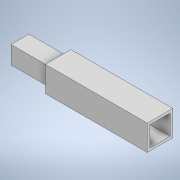
# Autodesk Inventor part: Right Side Piece
Saved by Autodesk Inventor 2022 (Build 260153000, 153)
## iProperties
Created: 2022-01-02
Part Number: Right Side Piece
Material: Generic
Document SubType Name: Modeling
Designer: josephinew
Density: 1 g/cm^3
Appearance: Default
Author: josephinew
Autodesk Inventor part; units mm, degrees
ref_plane "YZ Plane" through (0, 0, 0) normal (1, 0, 0) x (0, 1, 0)
ref_plane "XZ Plane" through (0, 0, 0) normal (0, 1, 0) x (-1, 0, 0)
ref_plane "XY Plane" through (0, 0, 0) normal (0, 0, 1) x (1, 0, 0)
sketch "Sketch1" plane through (0, 0, 0) normal (1, 0, 0) x (0, 1, 0)
  line L0 (0, 0) -> (25.4, 0)
  line L1 (25.4, 0) -> (25.4, -25.4)
  line L2 (25.4, -25.4) -> (0, -25.4)
  line L3 (0, -25.4) -> (0, 0)
  line L4 (0, 0) -> (3.175, 0)
  line L5 (0, -3.175) -> (0, 0)
  line L6 (3.175, -3.175) -> (22.225, -3.175)
  line L7 (22.225, -3.175) -> (22.225, -22.225)
  line L8 (22.225, -22.225) -> (3.175, -22.225)
  line L9 (3.175, -22.225) -> (3.175, -3.175)
  dimension "d0" = 25.4
  dimension "d1" = 25.4
  dimension "d6" = 19.05
  dimension "d7" = 19.05
  constraints: 20 end point, 4 parallel, 3 horizontal, 2 perpendicular
  measures "d0" distance of L1.end L2.end
  measures "d1" distance of L0.end L1.end
  measures "d6" distance of L7.end L8.end
  measures "d7" distance of L6.end L7.end
extrude "Extrusion1" add sketch "Sketch1" along normal blind 101.6 contours L0 L1 L2 L3 | L6 L7 L8 L9
sketch "Sketch2" plane through (101.6, 0, 0) normal (1, 0, 0) x (0, 0, -1)
  line L0 (22.733, 22.225) -> (22.733, 22.733)
  line L1 (22.733, 22.733) -> (22.225, 22.733)
  line L2 (2.667, 3.175) -> (2.667, 2.667)
  line L3 (2.667, 2.667) -> (3.175, 2.667)
  line L4 (2.667, 2.667) -> (22.733, 2.667)
  line L5 (22.733, 2.667) -> (22.733, 22.733)
  line L6 (22.733, 22.733) -> (2.667, 22.733)
  line L7 (2.667, 22.733) -> (2.667, 2.667)
  point P0 (0, 0)
  constraints: 16 end point, 2 parallel, 1 horizontal, 1 perpendicular
extrude "Extrusion2" cut sketch "Sketch2" against normal blind 50.8
sketch "Sketch3" plane through (0, 0, 0) normal (-1, 0, 0) x (0, 0, 1)
  line L0 (-25.4, 0) -> (-21.6315, 0)
  line L1 (-21.6315, 3.81) -> (-17.78, 3.81)
  line L2 (-21.6315, 7.62) -> (-21.6315, 3.81)
  line L3 (-3.81, 21.59) -> (-7.62, 21.59)
  line L4 (-3.81, 17.78) -> (-3.81, 21.59)
  line L5 (-21.6315, 3.81) -> (-3.81, 3.81)
  line L6 (-3.81, 3.81) -> (-3.81, 21.59)
  line L7 (-3.81, 21.59) -> (-21.6315, 21.59)
  line L8 (-21.6315, 21.59) -> (-21.6315, 3.81)
  line L9 (-17.8215, 7.6198) -> (-7.62, 7.6198)
  line L10 (-7.62, 7.6198) -> (-7.62, 17.78)
  line L11 (-7.62, 17.78) -> (-17.8215, 17.78)
  line L12 (-17.8215, 17.78) -> (-17.8215, 7.6198)
  point P0 (0, 25.4)
  constraints: 26 end point, 5 horizontal, 4 parallel, 2 perpendicular
extrude "Extrusion3" add sketch "Sketch3" along normal blind 38.1
body "Solid1"
